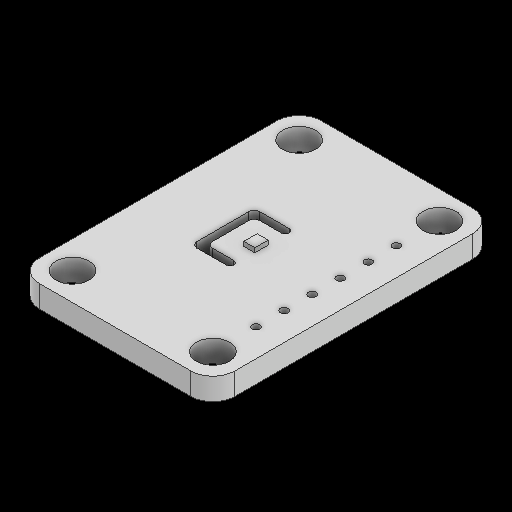
# Autodesk Inventor part: Temp_Basis_Platte
Saved by Autodesk Inventor 2027.1 (Build 311270010, 270A)
## iProperties
Created: 2026-10-08
Part Number: Temp_Basis_Platte
Material: Generisch
Document SubType Name: Modeling
Designer: josia
Density: 1 g/cm^3
Appearance: Vorgabe
Author: josia
Autodesk Inventor part; units mm, degrees
ref_plane "YZ Plane" through (0, 0, 0) normal (1, 0, 0) x (0, 1, 0)
ref_plane "XZ Plane" through (0, 0, 0) normal (0, 1, 0) x (-1, 0, 0)
ref_plane "XY Plane" through (0, 0, 0) normal (0, 0, 1) x (1, 0, 0)
sketch "Skizze1" plane through (0, 0, 0) normal (0, 1, 0) x (-1, 0, 0)
  line L0 (-8.85, -12.75) -> (8.85, -12.75)
  line L1 (8.85, -12.75) -> (8.85, 12.75)
  line L2 (8.85, 12.75) -> (-8.85, 12.75)
  line L3 (-8.85, 12.75) -> (-8.85, -12.75)
  line L4 (-8.85, -12.75) -> (8.85, 12.75) construction
  line L5 (8.85, -12.75) -> (-8.85, 12.75) construction
  point P0 (0, 0)
  dimension "d0" = 17.7
  dimension "d1" = 25.5
  constraints: 12 end point, 2 midpoint, 2 parallel, 1 horizontal, 1 perpendicular
  measures "d0" distance of L2.end L1.end
  measures "d1" distance of L1.end L0.end
extrude "Extrusion1" add sketch "Skizze1" along normal blind 2
fillet "Rundung1" radius 2 4 edges at (-8.85, 1, 12.75) (8.85, 1, 12.75) (8.85, 1, -12.75) (-8.85, 1, -12.75)
sketch "Skizze3" plane through (0, 2, 0) normal (0, 1, 0) x (1, 0, 0)
  line L0 (6.35, 10.25) -> (-6.35, 10.25)
  line L1 (-6.35, 10.25) -> (-6.35, -10.25)
  line L2 (-6.35, -10.25) -> (6.35, -10.25)
  line L3 (6.35, -10.25) -> (6.35, 10.25)
  line L4 (6.35, 10.25) -> (-6.35, -10.25) construction
  line L5 (-6.35, 10.25) -> (6.35, -10.25) construction
  line L6 (6.85, 12.75) -> (-6.85, 12.75) projected
  line L7 (-8.85, 10.75) -> (-8.85, -10.75) projected
  circle A0 centre (-6.35, 10.25) radius 1.5
  circle A1 centre (6.35, 10.25) radius 1.5
  circle A2 centre (6.35, -10.25) radius 1.5
  circle A3 centre (-6.35, -10.25) radius 1.5
  point P0 (0, 0)
  dimension "d16" = 2.5
  dimension "d17" = 2.5
  dimension "d18" = 3
  dimension "d19" = 3
  dimension "d20" = 3
  dimension "d21" = 3
  constraints: 12 end point, 4 centre point, 4 coincident, 2 midpoint, 2 parallel, 1 horizontal, 1 perpendicular
  measures "d16" distance between parallel lines of L7 L1
  measures "d17" distance between parallel lines of L6 L0
  measures "d18" diameter of A0
  measures "d19" diameter of A1
  measures "d20" diameter of A2
  measures "d21" diameter of A3
extrude "Extrusion2" cut sketch "Skizze3" against normal blind 3 contours A0 L1 L0 | L0 L1 A0 | A1 L3 L0 | L0 L3 A1 | A3 L2 L1 | L1 L2 A3 | A2 L2 L3 | L3 L2 A2
sketch "Skizze4" plane through (0, 2, 0) normal (0, 1, 0) x (1, 0, 0)
  circle A0 centre (6.35, -10.25) radius 1.5 projected
  circle A1 centre (6.35, 10.25) radius 1.5 projected
  line L0 (6.35, -10.25) -> (6.35, 10.25)
  circle A2 centre (6.35, -6.35) radius 0.35
  circle A3 centre (6.35, -3.81) radius 0.35
  circle A4 centre (6.35, -1.27) radius 0.35
  circle A5 centre (6.35, 1.27) radius 0.35
  circle A6 centre (6.35, 3.81) radius 0.35
  circle A7 centre (6.35, 6.35) radius 0.35
  point P0 (0, 0)
  point P1 (6.35, 0)
  dimension "d24" = 0.7
  dimension "d25" = 0.7
  dimension "d26" = 0.7
  dimension "d27" = 0.7
  dimension "d28" = 0.7
  dimension "d29" = 0.7
  dimension "d30" = 1.27
  dimension "d31" = 1.27
  dimension "d32" = 2.54
  dimension "d33" = 2.54
  dimension "d34" = 2.54
  dimension "d35" = 2.54
  constraints: 6 centre point, 10 other
  measures "d24" diameter of A2
  measures "d25" diameter of A3
  measures "d26" diameter of A4
  measures "d27" diameter of A5
  measures "d28" diameter of A6
  measures "d29" diameter of A7
  measures "d30" distance of point (6.35, 0) A4.centre
  measures "d31" distance of A5.centre point (6.35, 0)
  measures "d32" distance of A6.centre A5.centre
  measures "d33" distance of A6.centre A7.centre
  measures "d34" distance of A4.centre A3.centre
  measures "d35" distance of A3.centre A2.centre
extrude "Extrusion3" cut sketch "Skizze4" against normal blind 10 contours A2 L0 | L0 A2 | A3 L0 | L0 A3 | A4 L0 | L0 A4 | A5 L0 | L0 A5 | A6 L0 | L0 A6 | A7 L0 | L0 A7
sketch "Skizze5" plane through (0, 2, 0) normal (0, 1, 0) x (1, 0, 0)
  line L0 (-0.5, 0.6) -> (0.5, 0.6)
  line L1 (0.5, 0.6) -> (0.5, -0.6)
  line L2 (0.5, -0.6) -> (-0.5, -0.6)
  line L3 (-0.5, -0.6) -> (-0.5, 0.6)
  line L4 (-0.5, 0.6) -> (0.5, -0.6) construction
  line L5 (0.5, 0.6) -> (-0.5, -0.6) construction
  point P0 (0, 0)
  dimension "d38" = 1
  dimension "d39" = 1.2
  constraints: 12 end point, 2 midpoint, 2 parallel, 1 horizontal, 1 perpendicular
  measures "d38" distance of L1.end L2.end
  measures "d39" distance of L0.end L1.end
extrude "Extrusion4" add sketch "Skizze5" along normal blind 0.4
sketch "Skizze6" plane through (0, 2, 0) normal (0, 1, 0) x (1, 0, 0)
  line L0 (0, 0) -> (0, -2.5)
  line L1 (0, -2.5) -> (0, 2.5) construction
  line L2 (-0.5, -2.85) -> (0.5, -2.85)
  line L3 (0.5, -2.85) -> (0.5, -2.15)
  line L4 (0.5, -2.15) -> (-0.5, -2.15)
  line L5 (-0.5, -2.15) -> (-0.5, -2.85)
  line L6 (-0.5, -2.85) -> (0.5, -2.15) construction
  line L7 (0.5, -2.85) -> (-0.5, -2.15) construction
  line L8 (-0.5, 2.85) -> (0.5, 2.85)
  line L9 (0.5, 2.85) -> (0.5, 2.15)
  line L10 (0.5, 2.15) -> (-0.5, 2.15)
  line L11 (-0.5, 2.15) -> (-0.5, 2.85)
  line L12 (-0.5, 2.85) -> (0.5, 2.15) construction
  line L13 (0.5, 2.85) -> (-0.5, 2.15) construction
  line L14 (-0.5, -2.85) -> (-3, -2.85)
  line L15 (-3, -2.85) -> (-3, -2.15)
  line L16 (-3, -2.15) -> (-0.5, -2.15)
  line L17 (-0.5, -2.15) -> (-0.5, -2.85)
  line L18 (-0.5, 2.15) -> (-3, 2.15)
  line L19 (-3, 2.15) -> (-3, 2.85)
  line L20 (-3, 2.85) -> (-0.5, 2.85)
  line L21 (-0.5, 2.85) -> (-0.5, 2.15)
  line L22 (-3, -2.15) -> (-2.3, -2.15)
  line L23 (-2.3, -2.15) -> (-2.3, 2.15)
  line L24 (-2.3, 2.15) -> (-3, 2.15)
  line L25 (-3, 2.15) -> (-3, -2.15)
  point P0 (-2.3, -2.15)
  dimension "d44" = 2.5
  dimension "d45" = 5
  dimension "d46" = 0.7
  dimension "d47" = 0.7
  dimension "d48" = 2.5
  dimension "d49" = 0.7
  dimension "d55" = 0
  constraints: 52 end point, 10 parallel, 5 horizontal, 5 perpendicular, 4 midpoint, 4 point on line, 1 vertical
  measures "d44" distance of L0.start L0.end
  measures "d45" distance of L0.end L1.end
  measures "d46" distance of L3.end L2.end
  measures "d47" distance of L8.end L9.end
  measures "d48" distance of L15.end L16.end
  measures "d49" distance of L24.end L23.end
  measures "d55" distance between parallel lines of L8 L20
extrude "Extrusion5" cut sketch "Skizze6" against normal blind 10
fillet "Rundung4" radius 0.5 4 edges at (-3, 1, 2.85) (-2.3, 1, 2.15) (-3, 1, -2.85) (-2.3, 1, -2.15)
fillet "Rundung5" radius 0.35 4 edges at (0.5, 1, -2.85) (0.5, 1, -2.15) (0.5, 1, 2.15) (0.5, 1, 2.85)
equation "\"d22\" = d21"
